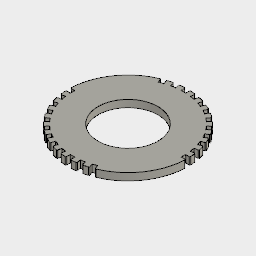
Top_v7 (Autodesk Fusion 360 design; units mm, degrees)
Autodesk Fusion 360 part; units mm, degrees
sketch "Sketch1" plane through (0, 0, 0) normal (0, 0, 1) x (1, 0, 0)
  circle A0 centre (0, 0) radius 20.5
  circle A1 centre (0, 0) radius 41
  line L0 (-38, -1.5) -> (-44, -1.5)
  line L1 (-44, -1.5) -> (-44, 1.5)
  line L2 (-44, 1.5) -> (-38, 1.5)
  line L3 (-38, 1.5) -> (-38, -1.5)
  line L4 (-38, -1.5) -> (-44, 1.5) construction
  line L5 (-44, -1.5) -> (-38, 1.5) construction
  circle A2 centre (0, 0) radius 28.25 construction
  line L6 (0, 0) -> (-41, 0) construction
  point P0 (-41, 0)
  dimension "d1" = 41
  dimension "d2" = 82
  dimension "d3" = 6
  dimension "d4" = 3
  dimension "d7" = 56.5
  measures "d1" diameter of A0
  measures "d2" diameter of A1
  measures "d3" distance of L1.end L2.end
  measures "d4" distance of L0.end L1.end
  measures "d7" diameter of A2
extrude "Extrude2" add sketch "Sketch1" along normal blind 5 contours A1 L0 L2 L3 picked at (-32.1154, -6.9726)
fillet "Fillet1" radius 0.5 2 edges at (-40.9726, 1.5, 2.5) (-40.9726, -1.5, 2.5)
pattern_circular "C-Pattern1" count 2 over 360 about axis through (0, 0, 1.75) along (0, 0, 1) of 5 faces at (-40.5482, 1.5096, 1.6667) (-39.6337, 1.5, 1.6667) (-38, 0.5, 1.6667) (-38.8169, -1.5, 1.6667) (-40.6863, -1.5591, 1.6667)
pattern_circular "C-Pattern2" count 12 over 110 about axis through (0, 0, 1.75) along (0, 0, 1) of 10 faces at (-40.5482, 1.5096, 1.6667) (-39.6337, 1.5, 1.6667) (-38, 0.5, 1.6667) (-38.8169, -1.5, 1.6667) (-40.6863, -1.5591, 1.6667) (40.5482, -1.5096, 1.6667) (39.6337, -1.5, 1.6667) (38, -0.5, 1.6667) (38.8169, 1.5, 1.6667) (40.6863, 1.5591, 1.6667)
